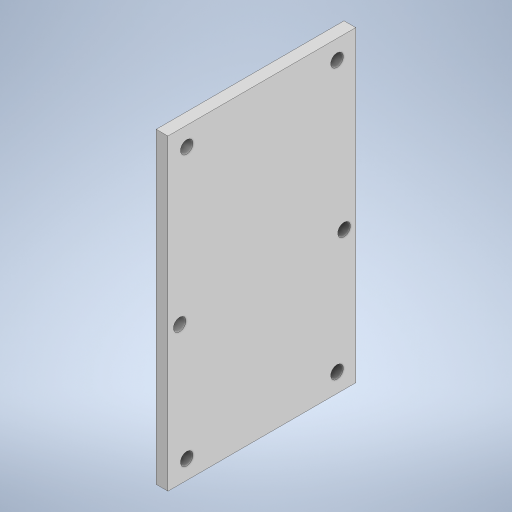
# Autodesk Inventor part: Engine Head Top
Saved by Autodesk Inventor 2023 (Build 270158000, 158)
## iProperties
Created: 2022-12-23
Part Number: Engine Head Top
Material: Generic
Document SubType Name: Modeling
Designer: tgr41
Density: 1 g/cm^3
Appearance: Default
Author: tgr41
Autodesk Inventor part; units mm, degrees
ref_plane "YZ Plane" through (0, 0, 0) normal (1, 0, 0) x (0, 1, 0)
ref_plane "XZ Plane" through (0, 0, 0) normal (0, 1, 0) x (-1, 0, 0)
ref_plane "XY Plane" through (0, 0, 0) normal (0, 0, 1) x (1, 0, 0)
sketch "Sketch1" plane through (0, 0, 0) normal (1, 0, 0) x (0, 1, 0)
  line L0 (0, 0) -> (83.185, 0)
  line L1 (83.185, 0) -> (83.185, -50.8)
  line L2 (83.185, -50.8) -> (0, -50.8)
  line L3 (0, -50.8) -> (0, 0)
  arc A0 (57.785, -44.45) -> (57.785, -6.35) centre (57.785, -25.4) ccw
  arc A1 (14.2875, -6.35) -> (6.35, -14.2875) centre (14.2875, -14.2875) ccw
  arc A2 (6.35, -36.5125) -> (14.2875, -44.45) centre (14.2875, -36.5125) ccw
  line L4 (14.2875, -44.45) -> (57.785, -44.45)
  line L5 (14.2875, -6.35) -> (57.785, -6.35)
  line L6 (6.35, -14.2875) -> (6.35, -36.5125)
  line L7 (57.785, 0) -> (57.785, -50.8)
  circle A3 centre (37.465, -3.175) radius 1.7145
  circle A4 centre (37.465, -47.625) radius 1.7145
  circle A5 centre (5.08, -45.72) radius 1.7145
  circle A6 centre (5.08, -5.08) radius 1.7145
  circle A7 centre (78.105, -5.08) radius 1.7145
  circle A8 centre (78.105, -45.72) radius 1.7145
  dimension "d0" = 83.185
  dimension "d1" = 50.8
  dimension "d2" = 38.1
  dimension "d3" = 25.4
  dimension "d4" = 25.4
  dimension "d5" = 15.875
  dimension "d6" = 15.875
  dimension "d7" = 14.2875
  dimension "d8" = 14.2875
  dimension "d9" = 14.2875
  dimension "d10" = 14.2875
  dimension "d19" = 25.4
  dimension "d20" = 3.175
  dimension "d21" = 3.175
  dimension "d28" = 3.429
  dimension "d29" = 5.08
  dimension "d30" = 5.08
  dimension "d31" = 45.72
  dimension "d32" = 45.72
  dimension "d33" = 3.429
  dimension "d34" = 3.429
  dimension "d35" = 5.08
  dimension "d36" = 5.08
  dimension "d37" = 5.08
  dimension "d38" = 5.08
  dimension "d39" = 5.08
  dimension "d40" = 5.08
  constraints: 16 end point, 9 centre point, 6 point on circle, 3 tangent, 2 parallel, 2 perpendicular, 2 point on line, 1 horizontal
  measures "d0" distance of L1.end L2.end
  measures "d1" distance of L0.end L1.end
  measures "d2" diameter of A0
  measures "d3" distance from line of L1 A0.centre
  measures "d4" distance from line of L2 A0.centre
  measures "d5" diameter of A1
  measures "d6" diameter of A2
  measures "d7" distance from line of L3 A1.centre
  measures "d8" distance from line of L3 A2.centre
  measures "d9" distance from line of L2 A2.centre
  measures "d10" distance from line of L0 A1.centre
  measures "d19" distance of L0.end L7.start
  measures "d20" distance from line of L2 A4.centre
  measures "d21" distance from line of L0 A3.centre
  measures "d28" diameter of A5
  measures "d29" distance from line of L2 A5.centre
  measures "d30" distance from line of L3 A5.centre
  measures "d31" distance from line of L1 A4.centre
  measures "d32" distance from line of L1 A3.centre
  measures "d33" diameter of A7
  measures "d34" diameter of A8
  measures "d35" distance from line of L2 A8.centre
  measures "d36" distance from line of L1 A8.centre
  measures "d37" distance from line of L1 A7.centre
  measures "d38" distance from line of L0 A7.centre
  measures "d39" distance from line of L3 A6.centre
  measures "d40" distance from line of L0 A6.centre
extrude "Extrusion1" add sketch "Sketch1" against normal blind 3.175
body "Solid1"
